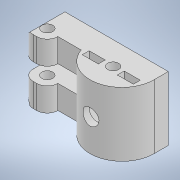
# Autodesk Inventor part: Деталь крепления диска к поворотному механизму
Saved by Autodesk Inventor 2020 (Build 240168000, 168)
## iProperties
Created: 2021-03-15
Part Number: Деталь крепления диска к поворотному механизму
Material: Типовые
Document SubType Name: Modeling
Designer: Антон
Density: 1 g/cm^3
Appearance: По умолчанию
Author: Антон
Autodesk Inventor part; units mm, degrees
ref_plane "YZ Plane" through (0, 0, 0) normal (1, 0, 0) x (0, 1, 0)
ref_plane "XZ Plane" through (0, 0, 0) normal (0, 1, 0) x (-1, 0, 0)
sketch "Эскиз1" plane through (0, 0, 0) normal (0, 0, 1) x (1, 0, 0)
  line L0 (0, 0) -> (18, 0)
  line L1 (18, 0) -> (18, 18)
  line L2 (18, 18) -> (0, 18)
  line L3 (0, 18) -> (0, 0)
  dimension "d0" = 18
  dimension "d1" = 18
  constraints: 8 end point, 2 parallel, 1 horizontal, 1 perpendicular
  measures "d0" distance of L2.end L1.end
  measures "d1" distance of L1.end L0.end
extrude "Выдавливание1" add sketch "Эскиз1" along normal blind 13
sketch "Эскиз2" plane through (0, 0, 0) normal (0, 0, -1) x (-1, 0, 0)
  line L0 (0, 0) -> (-18, 0) projected
  line L1 (-9, 0) -> (-9, 18)
  line L2 (-18, 18) -> (0, 18) projected
  circle A0 centre (-9, 9) radius 4.05
  dimension "d4" = 8.1
  constraints: 3 midpoint, 2 end point, 1 centre point
  measures "d4" diameter of A0
extrude "Выдавливание2" cut sketch "Эскиз2" against normal blind 11
sketch "Эскиз5" plane through (0, 18, 0) normal (0, 1, 0) x (1, 0, 0)
  line L0 (0, 0) -> (18, 0) projected
  line L1 (9, 0) -> (9, -6.5)
  circle A0 centre (9, -6.5) radius 1.55
  dimension "d21" = 6.5
  dimension "d22" = 3.1
  constraints: 2 end point, 1 centre point, 1 coincident, 1 midpoint, 1 vertical
  measures "d21" distance of L1.start L1.end
  measures "d22" diameter of A0
extrude "Выдавливание4" cut sketch "Эскиз5" against normal blind 4
sketch "Эскиз6" plane through (0, 0, 0) normal (0, -1, 0) x (1, 0, 0)
  circle A0 centre (9, 6.5) radius 1.55 projected
  point P0 (0, 0)
extrude "Выдавливание5" cut sketch "Эскиз6" against normal blind 4
sketch "Эскиз8" plane through (0, 0, 13) normal (0, 0, 1) x (1, 0, 0)
  circle A0 centre (9, 9) radius 4.05 projected
  circle A1 centre (9, 9) radius 4.05 projected
  circle A2 centre (9, 9) radius 2.25
  point P0 (0, 0)
  dimension "d27" = 4.5
  constraints: 1 centre point, 1 coincident
  measures "d27" diameter of A2
extrude "Выдавливание6" cut sketch "Эскиз8" against normal through all contours A2
sketch "Эскиз10" plane through (0, 0, 0) normal (-1, 0, 0) x (0, 0, 1)
  line L0 (0, 0) -> (0, 18) projected
  line L1 (0, 18) -> (7, 18)
  line L2 (7, 18) -> (7, 11.4)
  line L3 (7, 11.4) -> (0, 11.4)
  line L4 (0, 11.4) -> (0, 18)
  line L5 (0, 0) -> (7, 0)
  line L6 (7, 0) -> (7, 6.6)
  line L7 (7, 6.6) -> (0, 6.6)
  line L8 (0, 6.6) -> (0, 0)
  dimension "d39" = 7
  dimension "d40" = 6.6
  constraints: 16 end point, 4 parallel, 2 equal length, 2 horizontal, 2 perpendicular
  measures "d39" distance of L2.end L3.end
  measures "d40" distance of L1.end L2.end
extrude "Выдавливание8" add sketch "Эскиз10" along normal blind 13
ref_plane "РабПлоскость2" through (9, 0, 13) normal (-1, 0, 0) x (0, 0, 1)
sketch "Эскиз16" plane through (0, 11.4, 7) normal (0, 0, 1) x (1, 0, 0)
  line L0 (0, 6.6) -> (-13, 6.6) projected
  line L1 (0, 0) -> (-13, 0) projected
  line L2 (-13, 6.6) -> (-6, 6.6)
  line L3 (-6, 6.6) -> (-6, 0)
  line L4 (-6, 0) -> (-13, 0)
  line L5 (-13, 0) -> (-13, 6.6)
  line L6 (-13, -4.8) -> (-13, -11.4) projected
  line L7 (0, -11.4) -> (-13, -11.4) projected
  line L8 (-13, -4.8) -> (-6, -4.8)
  line L9 (-6, -4.8) -> (-6, -11.4)
  line L10 (-6, -11.4) -> (-13, -11.4)
  line L11 (-13, -11.4) -> (-13, -4.8)
  dimension "d50" = 7
  dimension "d51" = 7
  constraints: 16 end point, 4 parallel, 2 horizontal, 2 perpendicular, 2 point on line
  measures "d50" distance of L3.end L4.end
  measures "d51" distance of L9.end L10.end
extrude "Выдавливание10" add sketch "Эскиз16" along normal blind 3
sketch "Эскиз17" plane through (0, 18, 13) normal (0, 1, 0) x (1, 0, 0)
  line L0 (-6, 3) -> (-13, 3) projected
  line L1 (-9.5, 3) -> (-9.5, 20)
  circle A0 centre (9, 6.5) radius 1.55 projected
  line L2 (9, 6.5) -> (-9.5, 6.5)
  point P0 (0, 13)
  constraints: 4 end point, 1 midpoint, 1 perpendicular, 1 point on line, 1 vertical
hole "Отверстие2" at (-9.5, 18, 6.5) direction (0, -1, 0) diameter 3.1 end through all
mirror "Зеркальное отражение2" [suppressed]
fillet "Сопряжение8" radius 9 2 edges at (18, 9, 13) (0, 9, 13)
chamfer "Фаска2" distance 1.95 angle 45 2 edges at (-13, 18, 5) (-13, 0, 5)
fillet "Сопряжение12" radius 3 4 edges at (-13, 13.725, 10) (-13, 4.275, 10) (-6, 3.3, 10) (-6, 14.7, 10)
sketch "Эскиз19" plane through (0, 0, 0) normal (0, 0, -1) x (-1, 0, 0)
  circle A0 centre (-9, 9) radius 4.05 projected
  line L0 (-18, 0) -> (-18, 18) projected
  line L1 (-18, 18) -> (-11.8638, 11.8638)
  line L2 (0, 0) -> (-6.1362, 6.1362)
  line L3 (-0.5147, 0) -> (-18, 0) projected
  line L4 (-18, 0) -> (-11.8638, 6.1362)
  line L5 (0, 18) -> (-6.1362, 11.8638)
  line L6 (0, 0) -> (0, 18)
  line L7 (-18, 18) -> (11.05, 18) projected
  line L8 (11.05, 0) -> (-18, 0) projected
  line L9 (-14.9319, 14.9319) -> (-13.9319, 14.9319)
  line L10 (-3.0681, 14.9319) -> (-4.0681, 14.9319)
  line L11 (-14.9319, 3.0681) -> (-13.9319, 3.0681)
  line L12 (-3.0681, 3.0681) -> (-4.0681, 3.0681)
  dimension "d83" = 1
  constraints: 18 end point, 4 horizontal, 4 midpoint, 4 point on circle, 3 equal length, 2 collinear, 1 perpendicular, 1 point on line
  measures "d83" distance of L9.start L9.end
hole "Отверстие3" at (13.9319, 14.9319, 0) at (13.9319, 3.0681, 0) at (4.0681, 3.0681, 0) at (4.0681, 14.9319, 0) direction (0, 0, 1) diameter 2.2 depth 6.05
sketch "Эскиз21" plane through (0, 0, 0) normal (0, 0, -1) x (-1, 0, 0)
  circle A0 centre (-13.9319, 14.9319) radius 1.1
  line L0 (-12.8061, 16.8819) -> (-11.6802, 14.9319)
  line L1 (-11.6802, 14.9319) -> (-12.8061, 12.9819)
  line L2 (-12.8061, 12.9819) -> (-15.0577, 12.9819)
  line L3 (-15.0577, 12.9819) -> (-16.1836, 14.9319)
  line L4 (-16.1836, 14.9319) -> (-15.0577, 16.8819)
  line L5 (-15.0577, 16.8819) -> (-12.8061, 16.8819)
  line L6 (-16.1836, 14.9319) -> (-11.6802, 14.9319)
  line L7 (-11.6802, 14.9319) -> (-11.6802, 18)
  line L8 (-11.6802, 18) -> (-16.1836, 18)
  line L9 (-16.1836, 18) -> (-16.1836, 14.9319)
  line L10 (-18, 18) -> (11.05, 18) projected
  circle A1 centre (-13.9319, 14.9319) radius 1.1 projected
  line L11 (-10.55, 18) -> (-7.45, 18) projected
  line L12 (-9, 18) -> (-9, 0)
  line L13 (-18, 0) -> (-18, 18) projected
  line L14 (-18, 9) -> (0, 9)
  line L15 (0, 11.4) -> (0, 6.6) projected
  line L16 (-6.3198, 14.9319) -> (-5.1939, 12.9819)
  line L17 (-5.1939, 12.9819) -> (-2.9423, 12.9819)
  line L18 (-2.9423, 12.9819) -> (-1.8164, 14.9319)
  line L19 (-6.3198, 14.9319) -> (-6.3198, 18)
  line L20 (-6.3198, 18) -> (-1.8164, 18)
  line L21 (-1.8164, 18) -> (-1.8164, 14.9319)
  line L22 (-11.6802, 3.0681) -> (-12.8061, 5.0181)
  line L23 (-12.8061, 5.0181) -> (-15.0577, 5.0181)
  line L24 (-15.0577, 5.0181) -> (-16.1836, 3.0681)
  line L25 (-11.6802, 3.0681) -> (-11.6802, 0)
  line L26 (-11.6802, 0) -> (-16.1836, 0)
  line L27 (-16.1836, 0) -> (-16.1836, 3.0681)
  line L28 (-1.8164, 0) -> (-1.8164, 3.0681)
  line L29 (-6.3198, 0) -> (-1.8164, 0)
  line L30 (-6.3198, 3.0681) -> (-6.3198, 0)
  line L31 (-6.3198, 3.0681) -> (-5.1939, 5.0181)
  line L32 (-5.1939, 5.0181) -> (-2.9423, 5.0181)
  line L33 (-2.9423, 5.0181) -> (-1.8164, 3.0681)
  point P0 (-13.9319, 18)
  dimension "d84" = 3.9
  constraints: 60 end point, 18 symmetric about line, 5 midpoint, 2 coincident, 2 parallel, 1 centre point, 1 collinear, 1 concentric, 1 horizontal, 1 perpendicular, 1 vertical, 13 other
  measures "d84" distance between parallel lines of L2 L5
extrude "Выдавливание12" cut sketch "Эскиз21" against normal blind 1.95 from surface at -6.05 contours L6 A0 | L6 L1 L2 L3 A0 | A0 L6 L4 L5 L0 | A0 L6 | L0 L5 L4 L9 L8 L7 | L10 L21 L18 L17 L16 L19 | L25 L26 L27 L24 L23 L22 | L29 L30 L31 L32 L33 L28
equation "\"d51\" = d50"
